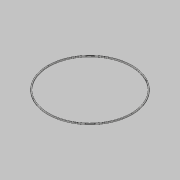
# Autodesk Inventor part: FeedHoop37
Saved by Autodesk Inventor 2017 (Build 210142000, 142)
## iProperties
Created: 2016-10-11
Part Number: FeedHoop37
Material: Generic
Document SubType Name: Modeling
Designer: krosie
Density: 1 g/cm^3
Appearance: Default
Author: krosie
Autodesk Inventor part; units mm, degrees
ref_plane "YZ Plane" through (0, 0, 0) normal (1, 0, 0) x (0, 1, 0)
ref_plane "XZ Plane" through (0, 0, 0) normal (0, 1, 0) x (-1, 0, 0)
ref_plane "XY Plane" through (0, 0, 0) normal (0, 0, 1) x (1, 0, 0)
sketch "Sketch1" plane through (0, 0, 0) normal (0, 1, 0) x (-1, 0, 0)
  line L0 (860, 0) -> (-860, 0) construction
  line L1 (429.9968, 744.7763) -> (-397.0343, -687.6836) construction
  line L2 (-430, 744.7818) -> (430, -744.7818) construction
  circle A0 centre (0, 0) radius 856
  circle A1 centre (423.25, 733.0905) radius 4
  circle A2 centre (0, 0) radius 846.5 construction
  circle A3 centre (-423.25, 733.0905) radius 4
  circle A4 centre (-846.5, 0) radius 4
  circle A5 centre (-423.25, -733.0905) radius 4
  circle A6 centre (423.25, -733.0905) radius 4
  circle A7 centre (846.5, 0) radius 4
  dimension "d1" = 60
  dimension "d2" = 60
  dimension "d28" = 8
  dimension "d29" = 9.5
  dimension "d32" = 360
  constraints: 7 centre point, 6 end point, 3 midpoint, 2 coincident, 2 point on line, 1 horizontal, 16 other
  measures "d1" angle of L0 L1
  measures "d2" angle of L2 L1
  measures "d28" diameter of A1
sketch "Sketch2" plane through (0, 0, 0) normal (0, 0, 1) x (1, 0, 0)
  line L0 (860, 0) -> (-860, 0) construction
  line L1 (846.5, 0) -> (-846.5, 0) construction
  line L2 (837.25, -9.5) -> (855.75, -9.5)
  line L3 (856, -9.25) -> (856, 9.25)
  line L4 (855.75, 9.5) -> (837.25, 9.5)
  line L5 (837, 9.25) -> (837, -9.25)
  line L6 (837, -9.5) -> (856, 9.5) construction
  line L7 (856, -9.5) -> (837, 9.5) construction
  arc A0 (856, 9.25) -> (855.75, 9.5) centre (855.75, 9.25) ccw
  arc A1 (837.25, 9.5) -> (837, 9.25) centre (837.25, 9.25) ccw
  arc A2 (837, -9.25) -> (837.25, -9.5) centre (837.25, -9.25) ccw
  arc A3 (855.75, -9.5) -> (856, -9.25) centre (855.75, -9.25) ccw
  line L8 (838.85, 7.9) -> (854.15, 7.9)
  line L9 (854.4, 7.65) -> (854.4, -7.65)
  line L10 (854.15, -7.9) -> (838.85, -7.9)
  line L11 (838.6, -7.65) -> (838.6, 7.65)
  arc A4 (854.15, -7.9) -> (854.4, -7.65) centre (854.15, -7.65) ccw
  arc A5 (854.4, 7.65) -> (854.15, 7.9) centre (854.15, 7.65) ccw
  arc A6 (838.85, 7.9) -> (838.6, 7.65) centre (838.85, 7.65) ccw
  arc A7 (838.6, -7.65) -> (838.85, -7.9) centre (838.85, -7.65) ccw
  point P0 (0, 0)
  point P1 (850.5, 0)
  dimension "d34" = 19
  dimension "d35" = 19
  dimension "d36" = 0.25
  dimension "d37" = 1.6
  dimension "d38" = 0.25
  constraints: 20 end point, 16 point on circle, 16 tangent, 8 centre point, 8 point on line, 6 equal radius, 4 parallel, 2 midpoint, 2 perpendicular, 1 horizontal, 3 other
  measures "d34" distance of L7.end L6.end
  measures "d35" distance of L6.end L7.start
  measures "d36" radius of A0
  measures "d37" distance between parallel lines of L4 L8
  measures "d38" radius of A4
sweep "Sweep1" add profiles "Sketch2" path "Sketch1" path curves A0
extrude "Extrusion1" cut sketch "Sketch1" along normal through all both and the other way through all contours A1 | A3 | A4 | A5 | A6 | A7
body "Solid1"
